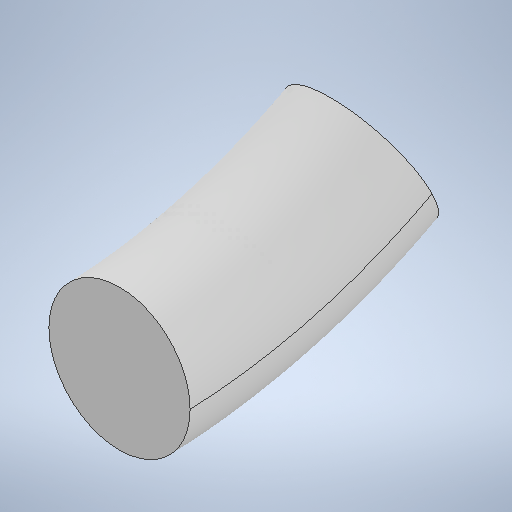
# Autodesk Inventor part: peca_009_001
Saved by Autodesk Inventor 2026 (Build 300175000, 175)
## iProperties
Created: 2025-03-26
Part Number: peca_009_001
Material: Generic
Document SubType Name: Modeling
Designer: Carlos Dias
Density: 1 g/cm^3
Appearance: Default
Author: Carlos Dias
Autodesk Inventor part; units mm, degrees
ref_plane "YZ Plane" through (0, 0, 0) normal (1, 0, 0) x (0, 1, 0)
ref_plane "XZ Plane" through (0, 0, 0) normal (0, 1, 0) x (-1, 0, 0)
ref_plane "XY Plane" through (0, 0, 0) normal (0, 0, 1) x (1, 0, 0)
sketch "Sketch2" plane through (0, 0, 0) normal (0, 0, 1) x (1, 0, 0)
  circle A0 centre (0, 0) radius 5.0467
  constraints: 1 centre point, 1 coincident
sketch "Sketch3" plane through (0, 0, 0) normal (1, 0, 0) x (0, 1, 0)
  arc A0 (0, 0) -> (4.6916, -17.3028) centre (39.7945, 1.5027) ccw
  constraints: 2 point on circle, 1 centre point
sweep "Sweep1" add profiles "Sketch2" path "Sketch3"
body "Solid1"
